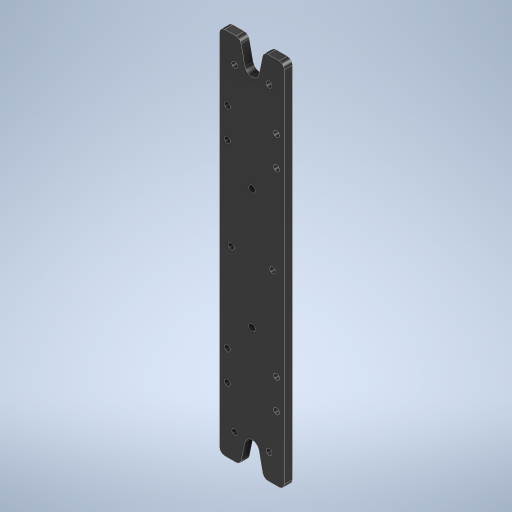
# Autodesk Inventor part: InitialPositioningFrame
Saved by Autodesk Inventor 2024.2 (Build 282272000, 272)
## iProperties
Created: 2024-01-11
Part Number: InitialPositioningFrame
Material: Aluminum 7075
Document SubType Name: Modeling
Designer: Masato Kubotera
Density: 2.81 g/cm^3
Appearance: Glossy - Black
Vendor: meviy
Mass: 301.604 g
Surface Area: 490.296 cm^2
Volume: 107.332 cm^3
Author: Masato Kubotera
Autodesk Inventor part; units mm, degrees
ref_plane "YZ Plane" through (0, 0, 0) normal (1, 0, 0) x (0, 1, 0)
ref_plane "XZ Plane" through (0, 0, 0) normal (0, 1, 0) x (-1, 0, 0)
ref_plane "XY Plane" through (0, 0, 0) normal (0, 0, 1) x (1, 0, 0)
sketch "Sketch1" plane through (0, 0, 0) normal (1, 0, 0) x (0, 1, 0)
  line L0 (31.625, -180) -> (-31.625, -180)
  line L1 (-31.625, -180) -> (-31.625, 180)
  line L2 (-31.625, 180) -> (31.625, 180)
  line L3 (31.625, 180) -> (31.625, -180)
  line L4 (31.625, -180) -> (-31.625, 180) construction
  line L5 (-31.625, -180) -> (31.625, 180) construction
  line L6 (-31.625, 0) -> (31.625, 0) construction
  line L7 (0, 180) -> (0, -180) construction
  line L8 (24, -88) -> (-24, -88) construction
  line L9 (24, -117) -> (-24, -117) construction
  line L10 (16.75, -155) -> (-16.75, -155) construction
  line L11 (24, 88) -> (-24, 88) construction
  line L12 (24, 117) -> (-24, 117) construction
  line L13 (16.75, 155) -> (-16.75, 155) construction
  line L14 (24, -117) -> (24, -88) construction
  arc A0 (-6.8516, 158.566) -> (6.8516, 158.566) centre (0, 160) ccw
  line L15 (-15, 197.5) -> (15, 197.5)
  line L16 (15, 197.5) -> (6.8516, 158.566)
  line L17 (-15, 197.5) -> (-6.8516, 158.566)
  arc A1 (6.8516, -158.566) -> (-6.8516, -158.566) centre (0, -160) ccw
  line L18 (-15, -197.5) -> (15, -197.5)
  line L19 (15, -197.5) -> (6.8516, -158.566)
  line L20 (-15, -197.5) -> (-6.8516, -158.566)
  point P0 (0, 0)
  point P1 (-20.25, 0)
  point P2 (20.25, 0)
  point P3 (0, 155)
  point P4 (-11.3374, -180)
  point P5 (11.3374, -180)
  point P6 (11.3374, 180)
  point P7 (-11.3374, 180)
  point P8 (0, 58.5)
  point P9 (0, -58.5)
  dimension "d0" = 63.25
  dimension "d1" = 360
  dimension "d2" = 40.5
  dimension "d3" = 176
  dimension "d4" = 29
  dimension "d5" = 48
  dimension "d6" = 33.5
  dimension "d7" = 310
  dimension "d8" = 30
  dimension "d9" = 37.5
  dimension "d10" = 14
  dimension "d11" = 320
  dimension "d21" = 117
  constraints: 42 end point, 22 symmetric about line, 8 coincident, 7 midpoint, 5 horizontal, 5 point on line, 4 point on circle, 2 centre point, 2 parallel, 1 perpendicular, 1 tangent, 1 vertical, 1 other
  measures "d0" distance of L1.end L2.end
  measures "d1" distance of L2.end L0.start
  measures "d2" distance of point (20.25, 0) point (-20.25, 0)
  measures "d3" distance between parallel lines of L8 L11
  measures "d4" distance of L9.start L8.start
  measures "d5" distance of L8.start L8.end
  measures "d6" distance of L10.start L10.end
  measures "d7" distance from line of point (0, 155) L10
  measures "d8" distance of L15.start L15.end
  measures "d9" distance from line of point (0, 160) L15
  measures "d10" diameter of A0
  measures "d11" distance of point (0, -160) point (0, 160)
  measures "d21" distance of point (0, -58.5) point (0, 58.5)
extrude "Extrusion1" add sketch "Sketch1" along normal blind 8 contours L0 L19 A1 L20 L1 L2 L17 A0 L16 L3
hole "Phi6-H7" at (0, -20.25, 0) at (0, 20.25, 0) at (0, 24, -88) at (0, 24, -117) at (0, 16.75, -155) at (0, -24, -88) at (0, -24, -117) at (0, -16.75, -155) at (0, 24, 88) at (0, 24, 117) at (0, 16.75, 155) at (0, -16.75, 155) at (0, -24, 117) at (0, -24, 88) at (0, 0, 160) at (0, 0, -160) direction (1, 0, 0) diameter 6 end through all
hole "M8" at (0, 0, 58.5) at (0, 0, -58.5) direction (1, 0, 0) diameter 6.647 end through all thread size "M8x1.25" class "6H" standard "ANSI Metric M Profile"
fillet "R5" radius 5 8 edges at (4, 31.625, 180) (4, -31.625, 180) (4, 31.625, -180) (4, 11.3374, -180) (4, -11.3374, -180) (4, -31.625, -180) (4, -11.3374, 180) (4, 11.3374, 180)
body "Solid1"
